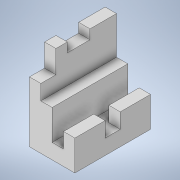
# Autodesk Inventor part: BT011
Saved by Autodesk Inventor 2022 (Build 260153000, 153)
## iProperties
Created: 2022-01-06
Part Number: BT011
Material: Generic
Document SubType Name: Modeling
Designer: Rayen
Density: 1 g/cm^3
Appearance: Default
Author: Rayen
Autodesk Inventor part; units mm, degrees
ref_plane "YZ Plane" through (0, 0, 0) normal (1, 0, 0) x (0, 1, 0)
ref_plane "XZ Plane" through (0, 0, 0) normal (0, 1, 0) x (-1, 0, 0)
sketch "Sketch1" plane through (0, 0, 0) normal (0, 0, 1) x (1, 0, 0)
  line L0 (-197.9412, -291.7647) -> (-197.9412, 108.2353)
  line L1 (-197.9412, 108.2353) -> (-97.9412, 108.2353)
  line L2 (-97.9412, 108.2353) -> (-97.9412, 258.2353)
  line L3 (-97.9412, 258.2353) -> (-22.9412, 258.2353)
  line L4 (-22.9412, 258.2353) -> (-22.9412, 195.8824)
  line L5 (-22.9412, 195.8824) -> (127.0588, 195.8824)
  line L6 (127.0588, 195.8824) -> (127.0588, 258.2353)
  line L7 (127.0588, 258.2353) -> (302.0588, 258.2353)
  line L8 (302.0588, 258.2353) -> (302.0588, -291.7647)
  line L9 (302.0588, -291.7647) -> (-197.9412, -291.7647)
  point P0 (0, 0)
  dimension "d0" = 100
  dimension "d1" = 75
  dimension "d2" = 150
  dimension "d3" = 500
  dimension "d4" = 400
  dimension "d5" = 550
  constraints: 20 end point, 8 perpendicular, 2 point on line, 1 vertical
  measures "d0" distance of L0.end L1.end
  measures "d1" distance of L2.end L3.end
  measures "d2" distance of L4.end L5.end
  measures "d3" distance of L8.end L0.start
  measures "d4" distance of L0.start L0.end
  measures "d5" distance of L7.end L8.end
extrude "Extrusion1" add sketch "Sketch1" along normal blind 75
sketch "Sketch2" plane through (0, 0, 75) normal (0, 0, 1) x (1, 0, 0)
  point P0 (0, 0)
ref_plane "Work Plane1" through (0, 0, 75) normal (0, 0, 1) x (1, 0, 0)
sketch "Sketch3" plane through (0, 0, 75) normal (0, 0, 1) x (1, 0, 0)
  line L0 (-197.9412, -291.7647) -> (-197.9412, 8.2353)
  line L1 (-197.9412, 8.2353) -> (302.0588, 8.2353)
  line L2 (302.0588, 8.2353) -> (302.0588, -291.7647)
  line L3 (302.0588, -291.7647) -> (-197.9412, -291.7647)
  line L4 (-197.9412, -291.7647) -> (302.0588, -291.7647) projected
  line L5 (-197.9412, 108.2353) -> (-197.9412, -291.7647) projected
  point P0 (0, 0)
  dimension "d9" = 300
  dimension "d10" = 500
  constraints: 8 end point, 3 collinear, 2 perpendicular, 1 vertical
  measures "d9" distance of L0.start L0.end
  measures "d10" distance of L2.end L0.start
extrude "Extrusion2" add sketch "Sketch3" along normal blind 75
ref_plane "Work Plane2" through (0, 0, 150) normal (0, 0, 1) x (1, 0, 0)
sketch "Sketch4" plane through (0, 0, 150) normal (0, 0, 1) x (1, 0, 0)
  line L0 (-197.9412, 108.2353) -> (-197.9412, -291.7647) projected
  line L1 (-197.9412, -191.7647) -> (302.0588, -191.7647)
  line L2 (302.0588, -291.7647) -> (302.0588, 258.2353) projected
  line L3 (-197.9412, -291.7647) -> (302.0588, -291.7647) projected
  point P0 (0, 0)
  dimension "d14" = 100
  constraints: 2 end point, 2 point on line, 1 horizontal
  measures "d14" distance between parallel lines of L3 L1
extrude "Extrusion3" add sketch "Sketch4" along normal blind 75
ref_plane "Work Plane3" through (0, 0, 225) normal (0, 0, 1) x (1, 0, 0)
sketch "Sketch5" plane through (0, 0, 225) normal (0, 0, 1) x (1, 0, 0)
  line L0 (-197.9412, 8.2353) -> (-197.9412, -191.7647) projected
  line L1 (-197.9412, -91.7647) -> (2.0588, -91.7647)
  line L2 (2.0588, -91.7647) -> (2.0588, -191.7647)
  line L3 (-197.9412, -191.7647) -> (302.0588, -191.7647) projected
  line L4 (102.0588, -191.7647) -> (102.0588, -91.7647)
  line L5 (102.0588, -91.7647) -> (302.0588, -91.7647)
  line L6 (302.0588, -191.7647) -> (-197.9412, -191.7647) projected
  line L7 (302.0588, -91.7647) -> (302.0588, -191.7647)
  line L8 (302.0588, -191.7647) -> (302.0588, -291.7647)
  line L9 (-197.9412, -291.7647) -> (302.0588, -291.7647) projected
  line L10 (302.0588, -291.7647) -> (-197.9412, -291.7647)
  line L11 (-197.9412, -291.7647) -> (-197.9412, -91.7647)
  line L12 (2.0588, -191.7647) -> (102.0588, -191.7647)
  point P0 (0, 0)
  dimension "d18" = 200
  dimension "d19" = 200
  dimension "d20" = 100
  dimension "d21" = 100
  constraints: 18 end point, 4 perpendicular, 4 point on line, 1 horizontal, 1 midpoint, 1 parallel
  measures "d18" distance of L1.start L1.end
  measures "d19" distance of L4.end L5.end
  measures "d20" distance of L1.end L2.end
  measures "d21" distance between parallel lines of L2 L4
extrude "Extrusion4" add sketch "Sketch5" along normal blind 75
body "Solid1"
